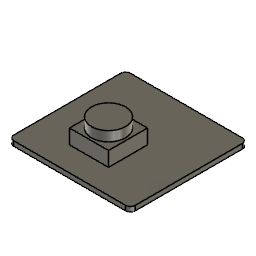
Camera (Autodesk Fusion 360 design; units mm, degrees)
Autodesk Fusion 360 part; units mm, degrees
sketch "Sketch1" plane through (0, 0, 0) normal (0, 0, 1) x (1, 0, 0)
  line L0 (12.5, -12) -> (-12.5, -12)
  line L1 (-12.5, -12) -> (-12.5, 12)
  line L2 (-12.5, 12) -> (12.5, 12)
  line L3 (12.5, 12) -> (12.5, -12)
  line L4 (12.5, -12) -> (-12.5, 12) construction
  line L5 (-12.5, -12) -> (12.5, 12) construction
  dimension "d1" = 25
  dimension "d2" = 24
  constraint horizontal L0
  constraint perpendicular L0 L1
  constraint parallel L0 L2
  constraint parallel L1 L3
  constraint coincident L4 origin
  constraint coincident L5 origin
  measures "d1" distance of L1.end L2.end
  measures "d2" distance of L0.end L1.end
extrude "Extrude1" add sketch "Sketch1" along normal blind 1
sketch "Sketch2" plane through (0, 0, 1) normal (0, 0, 1) x (-1, 0, 0)
  line L0 (-12.5, -12) -> (12.5, -12)
  line L1 (12.5, -12) -> (12.5, 12)
  line L2 (12.5, 12) -> (-12.5, 12)
  line L3 (-12.5, 12) -> (-12.5, -12)
  line L4 (5, 7) -> (-3, 7)
  line L5 (-3, 7) -> (-3, -1)
  line L6 (-3, -1) -> (5, -1)
  line L7 (5, -1) -> (5, 7)
  dimension "d5" = 8
  dimension "d6" = 8
  dimension "d7" = 7.5
  dimension "d8" = 5
  constraint horizontal L4
  constraint vertical L5
  constraint horizontal L6
  constraint vertical L7
  measures "d5" distance of L4.start L4.end
  measures "d6" distance of L4.start L6.end
  measures "d7" distance of L1 L7
  measures "d8" distance of L2 L4
extrude "Extrude2" add sketch "Sketch2" along normal blind 3 contours L4 L5 L6 L7
sketch "Sketch3" plane through (0, 0, 4) normal (0, 0, 1) x (-1, 0, 0)
  line L0 (5, -1) -> (5, 7)
  line L1 (5, 7) -> (-3, 7)
  line L2 (-3, 7) -> (-3, -1)
  line L3 (-3, -1) -> (5, -1)
  line L4 (-3, 3) -> (5, 3)
  line L5 (1, -1) -> (1, 7)
  circle A0 centre (1, 3) radius 3.5
  dimension "d11" = 7
  constraint midpoint L2 L4.start
  constraint midpoint L0 L4.end
  constraint midpoint L3 L5.start
  constraint midpoint L1 L5.end
  constraint midpoint L4 A0.centre
  measures "d11" diameter of A0
extrude "Extrude3" add sketch "Sketch3" along normal blind 2 contours L4 L5 A0 | L4 L5 A0 | L4 L5 A0 | L4 L5 A0
fillet "Fillet1" radius 1 4 edges at (-12.5, -12, 0.5) (12.5, 12, 0.5) (12.5, -12, 0.5) (-12.5, 12, 0.5)
